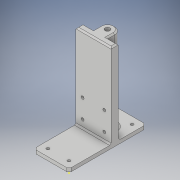
# Autodesk Inventor part: Part1
Saved by Autodesk Inventor 2019 (Build 230136000, 136)
## iProperties
Created: 2018-10-08
Part Number: Part1
Material: Generic
Document SubType Name: Modeling
Designer: Steven
Density: 1 g/cm^3
Appearance: Default
Author: Steven
Autodesk Inventor part; units mm, degrees
ref_plane "YZ Plane" through (0, 0, 0) normal (1, 0, 0) x (0, 1, 0)
ref_plane "XZ Plane" through (0, 0, 0) normal (0, 1, 0) x (-1, 0, 0)
ref_plane "XY Plane" through (0, 0, 0) normal (0, 0, 1) x (1, 0, 0)
sketch "Sketch1" plane through (0, 0, 0) normal (0, 1, 0) x (-1, 0, 0)
  point P0 (0, 0)
sketch "Sketch2" plane through (0, 0, 0) normal (0, 1, 0) x (-1, 0, 0)
  line L0 (0, 0) -> (50, 0)
  line L1 (50, 0) -> (50, -110)
  line L2 (50, -110) -> (0, -110)
  line L3 (0, -110) -> (0, 0)
  line L4 (25, 0) -> (25, -110) construction
  line L5 (50, -55) -> (0, -55) construction
  circle A0 centre (40, -10) radius 2
  circle A1 centre (40, -100) radius 2
  circle A2 centre (10, -10) radius 2
  circle A3 centre (10, -100) radius 2
  dimension "d0" = 50
  dimension "d1" = 110
  dimension "d2" = 4
  dimension "d3" = 10
  dimension "d4" = 10
  dimension "d7" = 90
  dimension "d10" = 30
  constraints: 12 end point, 4 centre point, 4 midpoint, 2 horizontal, 2 parallel, 1 perpendicular, 1 vertical, 6 other
  measures "d0" distance of L1.end L2.end
  measures "d1" distance of L0.end L1.end
  measures "d2" diameter of A0
  measures "d3" distance from line of L1 A0.centre
  measures "d4" distance from line of L0 A0.centre
  measures "d7" distance of A0.centre A1.centre
  measures "d10" distance of A0.centre A2.centre
extrude "Extrusion1" add sketch "Sketch2" along normal blind 5
sketch "Sketch3" plane through (0, 5, 0) normal (0, 1, 0) x (1, 0, 0)
  line L0 (-50, 110) -> (-50, 0) projected
  line L1 (0, 60) -> (-50, 60)
  line L2 (-50, 60) -> (-50, 70)
  line L3 (0, 70) -> (0, 60)
  line L4 (-50, 0) -> (0, 0) projected
  line L5 (0, 110) -> (-50, 110) construction
  line L6 (0, 0) -> (0, 110) projected
  circle A0 centre (-25, 80) radius 3.5
  arc A1 (-15, 80) -> (-35, 80) centre (-25, 80) ccw
  line L7 (-35, 80) -> (-35, 70)
  line L8 (-15, 80) -> (-15, 70)
  line L9 (-50, 70) -> (-35, 70)
  line L10 (-15, 70) -> (0, 70)
  dimension "d15" = 60
  dimension "d17" = 7
  dimension "d18" = 30
  constraints: 14 end point, 4 parallel, 3 perpendicular, 2 centre point, 2 point on circle, 1 coincident, 1 collinear, 1 horizontal, 1 point on line
  measures "d15" distance between parallel lines of L4 L1
  measures "d17" diameter of A0
  measures "d18" distance from line of L5 A0.centre
extrude "Extrusion2" add sketch "Sketch3" along normal blind 120 contours L9 L7 A1 L8 L10 L3 L1 L0
chamfer "Chamfer1" distance 2 angle 45 1 edges at (-25, 5, -60)
chamfer "Chamfer2" distance 3 angle 45 5 edges at (-7.5, 5, -70) (-42.5, 5, -70) (-25, 5, -90) (-15, 5, -75) (-35, 5, -75)
sketch "Sketch4" plane through (0, 125, -70) normal (0, 0, -1) x (-1, 0, 0)
  line L0 (0, 0) -> (15, 0) projected
  line L1 (15, -117) -> (0, -117) projected
  line L2 (35, 0) -> (50, 0) projected
  line L3 (50, -117) -> (35, -117) projected
  circle A0 centre (9.5, -109) radius 2
  circle A1 centre (40.5, -109) radius 2
  circle A2 centre (9.5, -82) radius 2
  circle A3 centre (40.5, -82) radius 2
  line L4 (0, -117) -> (0, 0) projected
  line L5 (50, -117) -> (50, 0) projected
  line L6 (0, -120) -> (50, -120) projected
  point P0 (0, -125)
  dimension "d27" = 4
  dimension "d29" = 4
  dimension "d31" = 4
  dimension "d32" = 4
  dimension "d33" = 27
  dimension "d34" = 27
  dimension "d35" = 9.5
  dimension "d36" = 9.5
  dimension "d37" = 9.5
  dimension "d38" = 9.5
  dimension "d40" = 11
  dimension "d41" = 11
  constraints: 4 centre point
  measures "d27" diameter of A0
  measures "d29" diameter of A1
  measures "d31" diameter of A2
  measures "d32" diameter of A3
  measures "d33" distance of A0.centre A2.centre
  measures "d34" distance of A1.centre A3.centre
  measures "d35" distance from line of L4 A0.centre
  measures "d36" distance from line of L4 A2.centre
  measures "d37" distance from line of L5 A3.centre
  measures "d38" distance from line of L5 A1.centre
  measures "d40" distance from line of L6 A0.centre
  measures "d41" distance from line of L6 A1.centre
extrude "Extrusion3" cut sketch "Sketch4" against normal blind 10
chamfer "Chamfer3" distance 2 angle 45 8 edges at (-25, 125, -90) (-35, 125, -75) (-15, 125, -75) (-7.5, 125, -70) (0, 125, -65) (-25, 125, -60) (-42.5, 125, -70) (-50, 125, -65)
chamfer "Chamfer4" distance 3 angle 45 4 edges at (0, 2.5, -110) (-50, 2.5, -110) (0, 2.5, 0) (-50, 2.5, 0)
body "Solid1"
